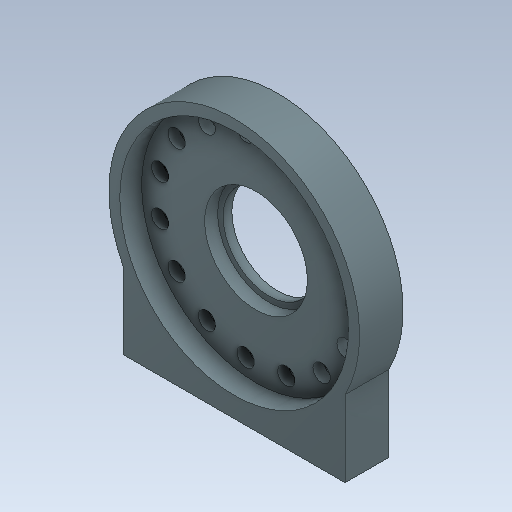
# Autodesk Inventor part: RearCover
Saved by Autodesk Inventor 2026.2 (Build 302298010, 298A)
## iProperties
Created: 2026-07-15
Part Number: RearCover
Material: Lead
Document SubType Name: Modeling
Designer: maxim
Density: 11.34 g/cm^3
Appearance: Lead
Author: maxim
Autodesk Inventor part; units mm, degrees
ref_plane "YZ Plane" through (0, 0, 0) normal (1, 0, 0) x (0, 1, 0)
ref_plane "XZ Plane" through (0, 0, 0) normal (0, 1, 0) x (-1, 0, 0)
ref_plane "XY Plane" through (0, 0, 0) normal (0, 0, 1) x (1, 0, 0)
sketch "Sketch1" plane through (0, 0, 0) normal (0, 0, 1) x (1, 0, 0)
  circle A0 centre (0, 0) radius 45 construction
  circle A1 centre (45, 0) radius 4
  circle A2 centre (0, 0) radius 52.5
  circle A3 centre (0, 0) radius 57.5
  circle A4 centre (0, 0) radius 23.6
  circle A5 centre (0, 0) radius 21.1
  line L0 (50.8901, -26.7665) -> (50.8901, -61.7665)
  line L1 (50.8901, -61.7665) -> (-50.8901, -61.7665)
  line L2 (-50.8901, -61.7665) -> (-50.8901, -26.7665)
  line L3 (12, -56.7665) -> (-20, -56.7665) construction
  dimension "d0" = 90
  dimension "d1" = 8
  dimension "d2" = 105
  dimension "d3" = 5
  dimension "d16" = 47.2
  dimension "d20" = 2.5
  dimension "d27" = 35
  dimension "d28" = 5
  constraints: 8 end point, 5 centre point, 4 coincident, 3 horizontal alignment, 2 perpendicular, 2 point on circle, 1 horizontal, 1 vertical, 2 other
  measures "d1" diameter of A1
  measures "d2" diameter of A2
  measures "d3" radial gap between concentric circles of A2 A3
  measures "d16" diameter of A4
  measures "d20" radial gap between concentric circles of A4 A5
  measures "d27" distance of L0.start L0.end
  measures "d28" distance between parallel lines of L1 L3
extrude "Extrusion1" add sketch "Sketch1" along normal blind 20 contours A3 | A3 L0 L1 L2
extrude "Extrusion2" add sketch "Sketch1" along normal blind 10 contours A1 | A2
extrude "Extrusion3" cut sketch "Sketch1" along normal through all contours A1
pattern_circular "Circular Pattern2" count 15 over 360 about axis through (0, 0, -10) along (0, 0, 1) of "Extrusion3"
extrude "Extrusion4" add sketch "Sketch1" along normal blind 4 contours A4
sketch "Sketch2" plane through (0, 0, 0) normal (0, 0, -1) x (1, 0, 0)
  circle A0 centre (-44.0166, -9.356) radius 7
  circle A1 centre (-44.0166, -9.356) radius 4 projected
  point P0 (0, 0)
  dimension "d21" = 14
  constraints: 1 centre point, 1 coincident
  measures "d21" diameter of A0
extrude "Extrusion5" cut sketch "Sketch2" against normal blind 5
pattern_circular "Circular Pattern3" count 15 over 360 about axis through (0, 0, 0) along (0, 0, 1) of "Extrusion5"
body "Solid1"
